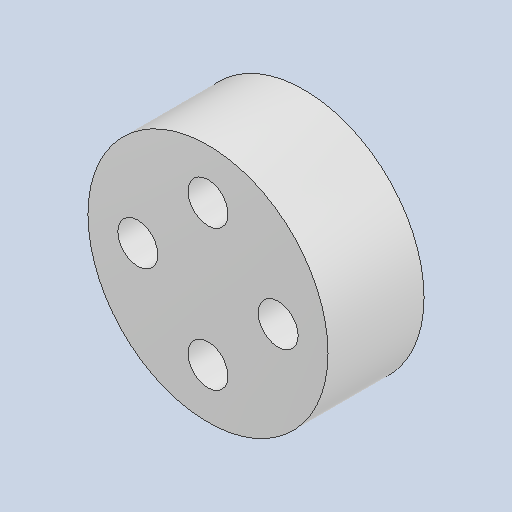
# Autodesk Inventor part: カム4
Saved by Autodesk Inventor 2023 (Build 270158030, 158C)
## iProperties
Created: 2021-09-27
Part Number: カム4
Material: Aluminum 2014-T6
Document SubType Name: Modeling
Designer: muzho
Density: 2.78927 g/cm^3
Appearance: Satin
Author: muzho
Autodesk Inventor part; units mm, degrees
ref_plane "YZ Plane" through (0, 0, 0) normal (1, 0, 0) x (0, 1, 0)
ref_plane "XZ Plane" through (0, 0, 0) normal (0, 1, 0) x (-1, 0, 0)
ref_plane "XY Plane" through (0, 0, 0) normal (0, 0, 1) x (1, 0, 0)
sketch "Sketch1" plane through (0, 0, 0) normal (0, 0, 1) x (1, 0, 0)
  circle A0 centre (0, 4.3841) radius 1.25
  circle A1 centre (-4.3841, 0) radius 1.25
  circle A2 centre (0, -4.3841) radius 1.25
  circle A3 centre (4.3841, 0) radius 1.25
  circle A4 centre (0, 0) radius 7.5
  dimension "d0" = 15
  constraints: 5 centre point, 2 coincident, 4 other
  measures "d0" diameter of A4
extrude "Extrusion1" add sketch "Sketch1" along normal blind 6
body "Solid1"
